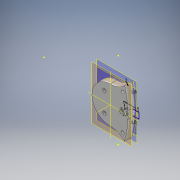
# Autodesk Inventor part: capacitor_glue
Saved by Autodesk Inventor 2019 (Build 230136000, 136)
## iProperties
Created: 2018-04-09
Part Number: capacitor_glue
Material: Générique
Document SubType Name: Modeling
Designer: Gregwar
Density: 1 g/cm^3
Appearance: Par défaut
Author: Gregwar
Autodesk Inventor part; units mm, degrees
ref_plane "YZ Plane" through (0, 0, 0) normal (1, 0, 0) x (0, 1, 0)
ref_plane "XZ Plane" through (0, 0, 0) normal (0, 1, 0) x (-1, 0, 0)
sketch "Esquisse1" plane through (0, 0, 0) normal (0, 1, 0) x (-1, 0, 0)
  circle A0 centre (0, 0) radius 17.75
  dimension "d0" = 35.5
  constraints: 1 centre point, 1 coincident
  measures "d0" diameter of A0
extrude "Extrusion1" add sketch "Esquisse1" along normal blind 8
ref_plane "Plan de construction1" through (0, 5, 0) normal (0, -1, 0) x (1, 0, 0)
sketch "Esquisse2" plane through (0, 5, 0) normal (0, -1, 0) x (1, 0, 0)
  circle A0 centre (0, 0) radius 17.75 construction
  line L0 (0, 0) -> (11, 0) construction
  circle A1 centre (11, 0) radius 1.65
  dimension "d4" = 11
  dimension "d5" = 3.3
  constraints: 2 end point, 1 centre point, 1 coincident, 1 horizontal
  measures "d4" distance of L0.start L0.end
  measures "d5" diameter of A1
extrude "Extrusion2" cut sketch "Esquisse2" along normal through all both and the other way through all
sketch "Esquisse3" plane through (0, 5, 0) normal (0, -1, 0) x (1, 0, 0)
  line L0 (23.2, 2.825) -> (8.2, 2.825)
  line L1 (8.2, 2.825) -> (8.2, -2.825)
  line L2 (8.2, -2.825) -> (23.2, -2.825)
  line L3 (23.2, -2.825) -> (23.2, 2.825)
  circle A0 centre (11, 0) radius 1.65 construction
  circle A1 centre (0, 0) radius 17.75 construction
  line L4 (0, 0) -> (8.2, 0) construction
  dimension "d8" = 5.65
  dimension "d9" = 2.8
  dimension "d10" = 15
  constraints: 10 end point, 2 horizontal, 2 parallel, 1 midpoint, 1 perpendicular
  measures "d8" distance of L0.end L1.end
  measures "d9" distance from line of A0.centre L1
  measures "d10" distance of L0.start L0.end
pattern_circular "Réseau circulaire1" count 3 over 360 about axis through (0, 0, 0) along (0, -1, 0) of "Extrusion2"
ref_plane "Work Plane2" through (0, 6.5, 0) normal (0, 1, 0) x (1, 0, 0)
sketch "Sketch4" plane through (0, 6.5, 0) normal (0, 1, 0) x (1, 0, 0)
  circle A0 centre (0, 0) radius 17
  circle A1 centre (-5.5, -9.5263) radius 1.65 projected
  circle A2 centre (11, 0) radius 1.65 projected
  circle A3 centre (0, 0) radius 17.75 projected
  circle A4 centre (0, 0) radius 17.75 projected
  line L0 (-5.1051, -17) -> (-5.1051, 17)
  dimension "d17" = 34
  constraints: 2 end point, 2 point on circle, 1 centre point, 1 coincident, 1 vertical
  measures "d17" diameter of A0
extrude "Extrusion4" [suppressed]
sketch "Sketch7" plane through (0, 0, 0) normal (0, -1, 0) x (1, 0, 0)
  circle A0 centre (-5.5, -9.5263) radius 1.65 projected
  circle A1 centre (-5.5, 9.5263) radius 1.65 projected
  circle A2 centre (11, 0) radius 1.65 projected
  circle A3 centre (0, 0) radius 17.75 projected
  arc A4 (12.2653, -21.0869) -> (-1.702, -23.304) centre (6.3902, -29.1791) ccw construction
  line L0 (12.2653, -21.0869) -> (14.1974, -23.6673) construction
  arc A5 (16.0148, -22.871) -> (19.1393, -21.699) centre (17.1898, -21.2525) ccw construction
  arc A6 (19.1393, -21.699) -> (17.9505, 23.1047) centre (-68.5898, -1.6093) ccw construction
  arc A7 (17.9505, 23.1047) -> (14.8221, 24.7813) centre (15.9506, 23.1301) ccw construction
  line L1 (14.8221, 24.7813) -> (14.299, 23.7665) construction
  circle A8 centre (10.9719, 0.0309) radius 1.5
  circle A9 centre (12.314, 17.2549) radius 1.5
  circle A10 centre (12.3141, -17.2245) radius 1.5
  circle A11 centre (10.9719, -0.0082) radius 3
  circle A12 centre (10.9719, -0.0082) radius 1.5
  circle A13 centre (12.3141, -17.2245) radius 1.5
  circle A14 centre (12.3141, -17.2245) radius 1.5
  arc A15 (14.1974, -23.6673) -> (17.3392, -3.7967) centre (-72.5704, 0.2356) ccw
  arc A16 (17.3635, 3.6841) -> (14.299, 23.7665) centre (-72.5704, 0.2356) ccw
  circle A17 centre (0, 0) radius 17.75 projected
  arc A18 (14.1974, -23.6673) -> (-0.0039, -17.75) centre (-0.0039, -37.75) ccw
  arc A19 (0, 17.75) -> (14.299, 23.7665) centre (0, 37.75) ccw
  circle A20 centre (-5.5, -9.5263) radius 1.65 projected
  circle A21 centre (-5.5, 9.5263) radius 1.65 projected
  circle A22 centre (11, 0) radius 1.65 projected
  circle A23 centre (0, 0) radius 17.75 projected
  dimension "d50" = 1.3141
  dimension "d51" = 17.2245
  dimension "d53" = 20
  dimension "d54" = 20
  dimension "d61" = 1.314
  dimension "d62" = 17.224
  dimension "d63" = 90
  dimension "d64" = 90
  dimension "d66" = 20
  dimension "d67" = 20
  constraints: 20 point on circle, 15 centre point, 4 end point, 2 coincident, 1 equal radius
  measures "d50" horizontal distance of A2.centre A10.centre
  measures "d51" vertical distance of A2.centre A10.centre
  measures "d53" radius of A18
  measures "d54" radius of A19
  measures "d61" horizontal distance of A2.centre A9.centre
  measures "d62" vertical distance of A9.centre A8.centre
  measures "d63" radius of A16
  measures "d64" radius of A15
  measures "d66" distance of A19.start A19.centre
  measures "d67" distance of A18.centre A18.end
extrude "Extrusion5" add sketch "Sketch7" against normal blind 8 contours A3 A19 A16 | A15 A18 A3
sketch "Sketch8" plane through (0, 8, 0) normal (0, 1, 0) x (1, 0, 0)
  circle A0 centre (12.3141, 17.2245) radius 1.5 projected
  circle A1 centre (12.314, -17.2549) radius 1.5 projected
  circle A2 centre (-5.5, 9.5263) radius 1.65 projected
  circle A3 centre (-5.5, -9.5263) radius 1.65 projected
  circle A4 centre (11, 0) radius 1.65 projected
  arc A5 (-0.0039, 17.75) -> (0, -17.75) centre (0, 0) ccw projected
  arc A6 (14.299, -23.7665) -> (0, -17.75) centre (0, -37.75) ccw projected
  arc A7 (14.299, -23.7665) -> (17.3635, -3.6841) centre (-72.5704, -0.2356) ccw projected
  arc A8 (17.3635, -3.6841) -> (17.3392, 3.7967) centre (0, 0) ccw projected
  arc A9 (17.3392, 3.7967) -> (14.1974, 23.6673) centre (-72.5704, -0.2356) ccw projected
  arc A10 (-0.0039, 17.75) -> (14.1974, 23.6673) centre (-0.0039, 37.75) ccw projected
  arc A11 (14.299, -23.7665) -> (0, -17.75) centre (0, -37.75) ccw projected
  arc A12 (14.8721, -21.5382) -> (13.3292, -20.2477) centre (0, -37.75) ccw
  arc A13 (12.6827, -1.3087) -> (12.7364, 0.5886) centre (0, 0) ccw
  arc A14 (10.3425, 14.4255) -> (10.6571, 14.5677) centre (-0.0039, 37.75) ccw
  arc A15 (15.5707, -3.4578) -> (15.5479, 3.5588) centre (0, 0) ccw
  arc A16 (15.5479, 3.5588) -> (13.2545, 20.0947) centre (-72.5704, -0.2356) ccw
  arc A17 (17.3392, 3.7967) -> (14.1974, 23.6673) centre (-72.5704, -0.2356) ccw projected
  arc A18 (13.3292, -20.2477) -> (15.5707, -3.4578) centre (-72.5704, -0.2356) ccw
  arc A19 (11.9075, 19.0825) -> (11.9222, 19.0926) centre (-0.6265, 37.1628) ccw
  arc A20 (13.2545, 20.0947) -> (14.7767, 21.4548) centre (-0.6265, 37.1628) ccw
  dimension "d59" = 2
  dimension "d68" = 1.8
  dimension "d69" = 1.8
  constraints: 19 point on circle, 8 centre point, 1 other
  measures "d59" radial gap between concentric circles of A6 A12
  measures "d68" radial gap between concentric circles of A7 A18
  measures "d69" radial gap between concentric circles of A16 A9
ref_plane "Work Plane3" through (0, 6.5, 0) normal (0, 1, 0) x (1, 0, 0)
ref_plane "Work Plane4" through (0, 1.5, 0) normal (0, -1, 0) x (1, 0, 0)
equation "\"d6\" = d5"
